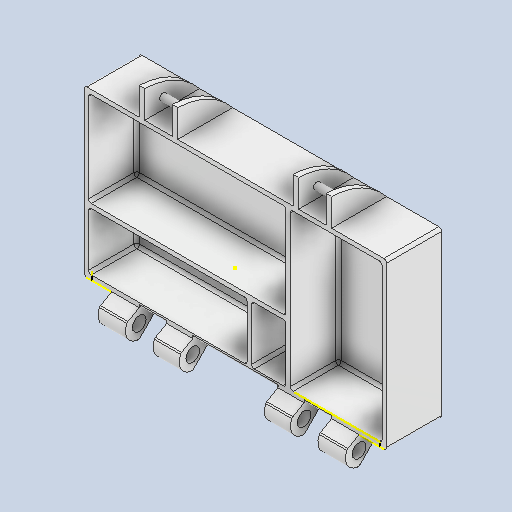
# Autodesk Inventor part: Scatola sotto
Saved by Autodesk Inventor 2023.2 (Build 272271030, 271C)
## iProperties
Created: 2023-02-07
Part Number: Scatola sotto
Material: Plastica ABS
Document SubType Name: Modeling
Designer: daler
Density: 1.06 g/cm^3
Appearance: Liscia - Bianco
Mass: 288.37 g
Surface Area: 1343.83 cm^2
Volume: 272.047 cm^3
Author: daler
Autodesk Inventor part; units mm, degrees
ref_plane "YZ Plane" through (0, 0, 0) normal (1, 0, 0) x (0, 1, 0)
ref_plane "XZ Plane" through (0, 0, 0) normal (0, 1, 0) x (-1, 0, 0)
ref_plane "XY Plane" through (0, 0, 0) normal (0, 0, 1) x (1, 0, 0)
sketch "Schizzo1" plane through (0, 0, 0) normal (0, 0, 1) x (1, 0, 0)
  line L0 (-110, 60) -> (110, 60)
  line L1 (110, 60) -> (110, -60)
  line L2 (110, -60) -> (-110, -60)
  line L3 (-110, -60) -> (-110, 60)
  line L4 (-110, 60) -> (110, -60) construction
  line L5 (110, 60) -> (-110, -60) construction
  line L6 (106.8, 56.8) -> (-106.8, 56.8)
  line L7 (-106.8, 56.8) -> (-106.8, -56.8)
  line L8 (-106.8, -56.8) -> (106.8, -56.8)
  line L9 (106.8, -56.8) -> (106.8, 56.8)
  point P0 (0, 0)
  point P1 (0, 0)
  dimension "d0" = 220
  dimension "d1" = 120
  dimension "d2" = 3.2
  constraints: 20 end point, 4 parallel, 2 perpendicular, 1 coincident, 1 horizontal, 1 midpoint, 3 other
  measures "d0" distance of L0.start L0.end
  measures "d1" distance of L0.end L1.end
  measures "d2" distance between parallel lines of L6 L0
extrude "Estrusione1" add sketch "Schizzo1" against normal blind 40 contours L0 L1 L2 L3 | L9 L8 L7 L6
extrude "Estrusione2" cut sketch "Schizzo1" against normal blind 35 contours L9 L8 L7 L6
sketch "Schizzo2" plane through (-110, -60, 0) normal (0, -1, 0) x (1, 0, 0)
  line L0 (220, 0) -> (0, 0) construction
  line L1 (20, 0) -> (20, -40) construction
  line L2 (0, -40) -> (220, -40) construction
  line L3 (110, 0) -> (110, -40) construction
  line L4 (0, 0) -> (0, -40) construction
  line L5 (40, 0) -> (40, -40) construction
  line L6 (60, 0) -> (60, -40) construction
  line L7 (79, 0) -> (79, -40) construction
  line L8 (20, 0) -> (40, 0)
  line L9 (40, 0) -> (40, -20)
  line L10 (40, -20) -> (20, -20)
  line L11 (20, -20) -> (20, 0)
  line L12 (60, 0) -> (79, 0)
  line L13 (79, 0) -> (79, -20)
  line L14 (79, -20) -> (60, -20)
  line L15 (60, -20) -> (60, 0)
  dimension "d7" = 20
  dimension "d8" = 20
  dimension "d9" = 20
  dimension "d10" = 19
  dimension "d11" = 20
  constraints: 26 end point, 9 point on line, 5 perpendicular, 4 parallel, 2 horizontal, 2 midpoint, 2 vertical
  measures "d7" distance between parallel lines of L4 L1
  measures "d8" distance between parallel lines of L5 L1
  measures "d9" distance between parallel lines of L6 L5
  measures "d10" distance between parallel lines of L7 L6
  measures "d11" distance between parallel lines of L10 L8
extrude "Estrusione3" add sketch "Schizzo2" along normal blind 20
sketch "Schizzo3" plane through (-31, -60, 0) normal (1, 0, 0) x (0, 0, -1)
  line L0 (0, 0) -> (40, 0) projected
  line L1 (0, -20) -> (20, -20) projected
  line L2 (20, 0) -> (0, -20)
  line L3 (20, -20) -> (20, 0)
  point P0 (0, 60)
  constraints: 4 end point, 1 midpoint, 1 vertical
extrude "Estrusione4" cut sketch "Schizzo3" against normal blind 100
sketch "Schizzo4" plane through (-31, -60, 0) normal (1, 0, 0) x (0, 0, -1)
  line L0 (0, 0) -> (0, -20) projected
  arc A0 (0, 0) -> (0, -20) centre (0, -10) ccw
  line L1 (0, -20) -> (0, 0)
  line L2 (0, 0) -> (20, 0) projected
  line L3 (0, 0) -> (-8.6391, -4.9635)
  point P0 (0, 60)
  constraints: 6 end point, 3 point on circle, 1 centre point, 1 collinear, 1 midpoint
extrude "Estrusione5" add sketch "Schizzo4" against normal blind 59
extrude "Estrusione6" cut sketch "Schizzo4" against normal blind 39
extrude "Estrusione7" add sketch "Schizzo4" against normal blind 19
sketch "Schizzo5" plane through (-31, -70, 0) normal (1, 0, 0) x (0, 0, -1)
  circle A0 centre (0, 0) radius 5
  arc A1 (0, 10) -> (0, -10) centre (0, 0) ccw projected
  point P0 (0, 70)
  dimension "d22" = 5
  dimension "d65" = 10
  constraints: 1 centre point
  measures "d22" radial gap between concentric circles of A1 A0
  measures "d65" diameter of A0
extrude "Estrusione8" cut sketch "Schizzo5" against normal blind 60
mirror "Specchio1" about plane through (0, 0, 0) normal (1, 0, 0) of "Estrusione8", "Estrusione7", "Estrusione6", "Estrusione5", "Estrusione4", "Estrusione3"
sketch "Schizzo7" plane through (0, 0, -40) normal (0, 0, -1) x (-1, 0, 0)
  line L0 (110, -60) -> (110, 60) projected
  line L1 (110, 60) -> (-40, 60)
  line L2 (-40, 60) -> (-40, -15)
  line L3 (-36.8, -15) -> (110, -15)
  line L4 (110, -15) -> (110, 60)
  line L5 (110, 60) -> (-36.8, 60)
  line L6 (-36.8, 60) -> (-36.8, -11.8)
  line L7 (-36.8, -11.8) -> (110, -11.8)
  line L8 (110, -11.8) -> (110, 60)
  line L9 (-40, -15) -> (-40, -56.8)
  line L10 (-50, -60) -> (-31, -60) projected
  line L11 (-36.8, -15) -> (-36.8, -56.8)
  line L12 (-106.8, -56.8) -> (106.8, -56.8) projected
  line L13 (-36.8, -56.8) -> (-40, -56.8)
  line L14 (-8.6, -15) -> (-8.6, -56.8)
  line L15 (-11.8, -15) -> (-11.8, -56.8)
  line L16 (-8.6, -56.8) -> (-11.8, -56.8)
  line L17 (110, -11.8) -> (110, -15)
  line L18 (-36.8, 60) -> (-40, 60)
  line L19 (110, 60) -> (-110, 60) projected
  point P0 (0, 0)
  point P1 (-36.8, -35.9)
  point P2 (-11.8, -35.9)
  point P3 (-36.8, 60)
  dimension "d37" = 150
  dimension "d38" = 75
  dimension "d39" = 3.2
  dimension "d40" = 3.2
  dimension "d41" = 3.2
  dimension "d42" = 41.8
  dimension "d43" = 3.2
  dimension "d44" = 25
  constraints: 32 end point, 6 point on line, 5 parallel, 5 perpendicular, 2 horizontal, 2 midpoint, 1 collinear, 1 vertical
  measures "d37" distance of L2.end L3.end
  measures "d38" distance of L1.end L2.end
  measures "d39" distance between parallel lines of L7 L3
  measures "d40" distance between parallel lines of L6 L2
  measures "d41" distance between parallel lines of L9 L11
  measures "d42" distance between parallel lines of L12 L3
  measures "d43" distance between parallel lines of L15 L14
  measures "d44" distance of point (-36.8, -35.9) point (-11.8, -35.9)
extrude "Estrusione9" add sketch "Schizzo7" against normal blind 40 contours L3 L11 L12 L9 L2 L1 L6 L7 L0 | L14 L12 L15 L3
sketch "Schizzo8" plane through (-110, 60, 0) normal (0, 1, 0) x (1, 0, 0)
  line L0 (180, 0) -> (180, 40) construction
  line L1 (0, 40) -> (220, 40) construction
  line L2 (176, 0) -> (176, 40) construction
  line L3 (220, 0) -> (220, 40) construction
  line L4 (156, 0) -> (156, 40) construction
  line L5 (152, 0) -> (152, 40) construction
  line L6 (176, 0) -> (180, 0)
  line L7 (180, 0) -> (180, 40)
  line L8 (180, 40) -> (176, 40)
  line L9 (176, 40) -> (176, 0)
  line L10 (156, 0) -> (152, 0)
  line L11 (152, 0) -> (152, 40)
  line L12 (152, 40) -> (156, 40)
  line L13 (156, 40) -> (156, 0)
  point P0 (110, 0)
  dimension "d47" = 40
  dimension "d48" = 4
  dimension "d49" = 20
  dimension "d50" = 4
  constraints: 24 end point, 5 parallel, 4 perpendicular, 4 point on line, 2 horizontal, 1 vertical
  measures "d47" distance between parallel lines of L0 L3
  measures "d48" distance between parallel lines of L2 L0
  measures "d49" distance between parallel lines of L2 L4
  measures "d50" distance between parallel lines of L5 L4
extrude "Estrusione10" add sketch "Schizzo8" along normal blind 20
sketch "Schizzo9" plane through (42, 60, -40) normal (-1, 0, 0) x (0, 0, 1)
  line L0 (40, 0) -> (40, 20) projected
  arc A0 (40, 20) -> (0, 0) centre (42.0137, -34.0274) ccw
  line L1 (0, 20) -> (40, 20) projected
  line L2 (40, 20) -> (0, 20)
  line L3 (0, 20) -> (0, 0)
  line L4 (40, 0) -> (40, 20) construction
  line L5 (40, 9.3852) -> (20, 0) construction
  line L6 (0, 0) -> (40, 0) construction
  line L7 (20, 15.3529) -> (20, 0) construction
  line L8 (20, 15.3529) -> (40, 9.3852) construction
  line L9 (20, 7.6764) -> (40, 9.3852) construction
  line L10 (30, 12.369) -> (20, 0) construction
  line L11 (30, 4.6926) -> (20, 15.3529) construction
  circle A1 centre (26.6667, 8.246) radius 2.5
  point P0 (40, -60)
  point P1 (0, 0)
  dimension "d55" = 5
  constraints: 16 end point, 4 midpoint, 3 point on circle, 3 point on line, 2 centre point, 1 collinear, 1 vertical
  measures "d55" diameter of A1
extrude "Estrusione11" cut sketch "Schizzo9" against normal blind 200 contours A0 L3 L1
extrude "Estrusione12" add sketch "Schizzo9" against normal up to next contours A1
mirror "Specchio2" about plane through (0, 0, 0) normal (1, 0, 0) of "Estrusione10", "Estrusione11", "Estrusione12"
fillet "Raccordo2" radius 2 46 edges at (-60, -60, 0) (60, -60, 0) (-80, -80, 0) (-40.5, -80, 0) (40.5, -80, 0) (80, -80, 0) (-80, -60, -20) (-40.5, -60, -20) (40.5, -60, -20) (80, -60, -20) (106.8, 56.8, -17.5) (106.8, 0, -35) (73.4, 56.8, -35) (106.8, -56.8, -17.5) (73.4, -56.8, -35) (36.8, 56.8, -17.5) (40, 56.8, -17.5) (40, 0, -35) (40, -56.8, -17.5) (11.8, -56.8, -17.5) (36.8, -56.8, -17.5) (11.8, -15, -17.5) (8.6, -15, -17.5) (36.8, -11.8, -17.5) (36.8, -15, -17.5) (11.8, -35.9, -35) (24.3, -56.8, -35) (24.3, -15, -35) (-35, -11.8, -35) (36.8, -35.9, -35) (36.8, 22.5, -35) (8.6, -35.9, -35) (8.6, -56.8, -17.5) (-49.1, -56.8, -35) (-49.1, -15, -35) (-106.8, -56.8, -17.5) (-106.8, -35.9, -35) (-106.8, -15, -17.5) (-106.8, -11.8, -17.5) (-106.8, 22.5, -35) (-106.8, 56.8, -17.5) (-35, 56.8, -35) (110, -60, -20) (-110, -60, -20) (-110, 60, -20) (110, 60, -20)
fillet "Raccordo3" radius 2 1 edges at (0, -60, 0)
sketch "Schizzo10" plane through (0, 0, 0) normal (0, 0, 1) x (1, 0, 0)
  line L0 (-104.8, -54.8) -> (-104.8, -56.8) projected
  line L1 (-104.8, -56.8) -> (-104.8, -60)
  line L2 (-108, -60) -> (-90, -60) projected
  line L3 (104.8, -56.8) -> (42, -56.8) projected
  line L4 (104.8, -56.8) -> (104.8, -60)
  line L5 (90, -60) -> (108, -60) projected
  point P0 (0, 0)
  constraints: 4 end point, 2 point on line, 2 vertical
extrude "Estrusione13" cut sketch "Schizzo4" along normal mid plane 1000 contours L3 A0
fillet "Raccordo5" radius 2 4 edges at (80, -64.9635, 8.6391) (40.5, -64.9635, 8.6391) (-40.5, -64.9635, 8.6391) (-80, -64.9635, 8.6391)
equation "\"d9\" = d8"
